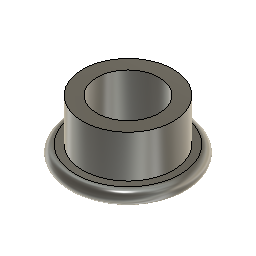
octopus ring thingy holder v3 (Autodesk Fusion 360 design; units mm, degrees)
Autodesk Fusion 360 part; units mm, degrees
sketch "Sketch1" plane through (0, 0, 0) normal (0, 0, 1) x (1, 0, 0)
  circle A0 centre (0, 0) radius 3.2
  dimension "d1" = 6.4
  constraint coincident A0.centre origin
  measures "d1" diameter of A0
extrude "Extrude1" add sketch "Sketch1" along normal blind 4 thin wall 1 inside makes body 1
copy_body "CopyPasteBodies1" bodies 1 makes body 2
move_body "Move1" bodies 2 to x (1, 0, 0) y (0, 1, 0) z (0, 0, 1) at (0, 0, 12)
move_face "OffsetFaces1" offset -3 1 faces at (2.8466, -0.2683, 16) on bodies 2
move_face "OffsetFaces2" offset 1 1 faces at (3.196, 0.1595, 12.3333) on bodies 2
move_face "OffsetFaces3" offset -1 1 faces at (2.1973, 0.1097, 12.3333) on bodies 2
fillet "Fillet1" radius 0.5 2 edges at (-3.9158, -1.5188, 13) (-3.9158, -1.5188, 12) on bodies 2
move_body "Move2" bodies 2 to x (1, 0, 0) y (0, 1, 0) z (0, 0, 1) at (0, 0, -12)
